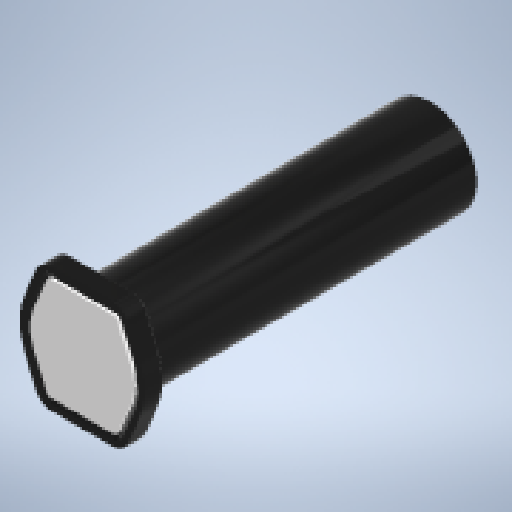
# Autodesk Inventor part: Spool Stud
Saved by Autodesk Inventor 2024 (Build 280153000, 153)
## iProperties
Created: 2025-01-02
Part Number: Spool Stud
Material: ABS Plastic
Document SubType Name: Modeling
Designer: Ishaan
Density: 1.06 g/cm^3
Appearance: Smooth - Black
Author: Ishaan
Autodesk Inventor part; units mm, degrees
ref_plane "YZ Plane" through (0, 0, 0) normal (1, 0, 0) x (0, 1, 0)
ref_plane "XZ Plane" through (0, 0, 0) normal (0, 1, 0) x (-1, 0, 0)
ref_plane "XY Plane" through (0, 0, 0) normal (0, 0, 1) x (1, 0, 0)
sketch "Sketch1" plane through (0, 0, 0) normal (0, 0, 1) x (1, 0, 0)
  circle A0 centre (0, 0) radius 15
  dimension "d0" = 30
  constraints: 1 centre point, 1 coincident
  measures "d0" diameter of A0
extrude "Extrusion1" add sketch "Sketch1" along normal blind 105
ref_plane "Work Plane1" through (0, 0, 8) normal (0, 0, -1) x (-1, 0, 0)
sketch "Sketch2" plane through (0, 0, 105) normal (0, 0, 1) x (1, 0, 0)
  line L0 (0, 7.5) -> (0, -7.5) construction
  point P0 (0, 0)
  point P1 (0, 0)
  dimension "d4" = 15
  constraints: 2 end point, 1 coincident, 1 midpoint, 1 vertical
  measures "d4" distance of L0.start L0.end
hole "Hole1" at (0, 7.5, 105) at (0, -7.5, 105) direction (0, 0, -1) diameter 10 depth 97
sketch "Sketch3" plane through (0, 7.5, 8) normal (0, 0, 1) x (1, 0, 0)
  circle A0 centre (0, 0) radius 5 projected
  circle A1 centre (0, -15) radius 5 projected
  point P0 (0, -7.5)
hole "Hole2" at (0, 7.5, 8) at (0, -7.5, 8) direction (0, 0, -1) diameter 5.4 end through all
sketch "Sketch4" plane through (0, 0, 105) normal (0, 0, 1) x (1, 0, 0)
  circle A0 centre (0, -7.5) radius 5 projected
  circle A1 centre (0, 7.5) radius 5 projected
  circle A2 centre (0, 0) radius 15 projected
  circle A3 centre (0, 0) radius 20
  line L0 (-18.4776, 7.6537) -> (-13.3636, 20)
  line L1 (-13.3636, 20) -> (13.3636, 20)
  line L2 (13.3636, 20) -> (18.4776, 7.6537)
  line L3 (18.4776, -7.6537) -> (13.3636, -20)
  line L4 (13.3636, -20) -> (-13.3636, -20)
  line L5 (-13.3636, -20) -> (-18.4776, -7.6537)
  dimension "d19" = 40
  dimension "d20" = 135
  dimension "d21" = 135
  constraints: 12 end point, 6 tangent, 4 point on circle, 2 horizontal, 2 vertical alignment, 1 centre point, 1 coincident
  measures "d19" diameter of A3
  measures "d20" angle of L3 L2
  measures "d21" angle of L5 L0
extrude "Extrusion2" add sketch "Sketch4" along normal blind 6.5 contours A2 | A3 | A3 L1 L2 | L3 L4 A3 | A3 L0 L1 | L4 L5 A3
fillet "Fillet1" radius 5 4 edges at (-13.3636, 20, 108.25) (-13.3636, -20, 108.25) (13.3636, -20, 108.25) (13.3636, 20, 108.25)
sketch "Sketch5" plane through (0, 0, 111.5) normal (0, 0, 1) x (1, 0, 0)
  arc A0 (14.6421, 16.9134) -> (10.0227, 20) centre (10.0227, 15) ccw projected
  line L0 (10.0227, 20) -> (-10.0227, 20) projected
  arc A1 (-10.0227, 20) -> (-14.6421, 16.9134) centre (-10.0227, 15) ccw projected
  line L1 (-14.6421, 16.9134) -> (-18.4776, 7.6537) projected
  arc A2 (-18.4776, 7.6537) -> (-18.4776, -7.6537) centre (0, 0) ccw projected
  line L2 (-18.4776, -7.6537) -> (-14.6421, -16.9134) projected
  arc A3 (-14.6421, -16.9134) -> (-10.0227, -20) centre (-10.0227, -15) ccw projected
  line L3 (-10.0227, -20) -> (10.0227, -20) projected
  arc A4 (10.0227, -20) -> (14.6421, -16.9134) centre (10.0227, -15) ccw projected
  line L4 (14.6421, -16.9134) -> (18.4776, -7.6537) projected
  arc A5 (18.4776, -7.6537) -> (18.4776, 7.6537) centre (0, 0) ccw projected
  line L5 (18.4776, 7.6537) -> (14.6421, 16.9134) projected
  circle A6 centre (0, 7.5) radius 5 projected
  circle A7 centre (0, -7.5) radius 5 projected
  line L6 (-10.0227, 18) -> (10.0227, 18)
  arc A8 (12.7943, 16.1481) -> (10.0227, 18) centre (10.0227, 15) ccw
  line L7 (12.7943, 16.1481) -> (16.6298, 6.8883)
  arc A9 (16.6298, -6.8883) -> (16.6298, 6.8883) centre (0, 0) ccw
  line L8 (16.6298, -6.8883) -> (12.7943, -16.1481)
  arc A10 (10.0227, -18) -> (12.7943, -16.1481) centre (10.0227, -15) ccw
  line L9 (10.0227, -18) -> (-10.0227, -18)
  arc A11 (-12.7943, -16.1481) -> (-10.0227, -18) centre (-10.0227, -15) ccw
  line L10 (-12.7943, -16.1481) -> (-16.6298, -6.8883)
  arc A12 (-16.6298, 6.8883) -> (-16.6298, -6.8883) centre (0, 0) ccw
  line L11 (-16.6298, 6.8883) -> (-12.7943, 16.1481)
  arc A13 (-10.0227, 18) -> (-12.7943, 16.1481) centre (-10.0227, 15) ccw
  dimension "d25" = 2
  constraints: 12 end point, 12 point on circle, 6 centre point, 11 other
  measures "d25" distance between parallel lines of L0 L6
extrude "Extrusion3" cut sketch "Sketch5" against normal blind 2.5 contours L6 A8 L7 A9 L8 A10 L9 A11 L10 A12 L11 A13
chamfer "Chamfer1" distance 2.5 angle 45 12 edges at (-14.7121, 11.5182, 109) (-11.6894, 17.4944, 109) (0, 18, 109) (11.6894, 17.4944, 109) (14.7121, 11.5182, 109) (18, 0, 109) (14.7121, -11.5182, 109) (11.6894, -17.4944, 109) (0, -18, 109) (-11.6894, -17.4944, 109) (-14.7121, -11.5182, 109) (-18, 0, 109)
ref_plane "Work Plane2" through (0, 0, 109.4) normal (0, 0, 1) x (1, 0, 0)
sketch "Sketch6" plane through (0, 0, 109) normal (0, 0, 1) x (1, 0, 0)
  circle A0 centre (0, 7.5) radius 5 projected
  circle A1 centre (0, -7.5) radius 5 projected
  line L0 (-14.3201, 5.9316) -> (-10.4846, 15.1913) projected
  arc A2 (-14.3201, 5.9316) -> (-14.3201, -5.9316) centre (0, 0) ccw projected
  line L1 (-10.4846, -15.1913) -> (-14.3201, -5.9316) projected
  arc A3 (-10.4846, -15.1913) -> (-10.0227, -15.5) centre (-10.0227, -15) ccw projected
  line L2 (10.0227, -15.5) -> (-10.0227, -15.5) projected
  arc A4 (10.0227, -15.5) -> (10.4846, -15.1913) centre (10.0227, -15) ccw projected
  line L3 (14.3201, -5.9316) -> (10.4846, -15.1913) projected
  arc A5 (14.3201, -5.9316) -> (14.3201, 5.9316) centre (0, 0) ccw projected
  line L4 (10.4846, 15.1913) -> (14.3201, 5.9316) projected
  arc A6 (10.4846, 15.1913) -> (10.0227, 15.5) centre (10.0227, 15) ccw projected
  line L5 (-10.0227, 15.5) -> (10.0227, 15.5) projected
  arc A7 (-10.0227, 15.5) -> (-10.4846, 15.1913) centre (-10.0227, 15) ccw projected
  arc A8 (11.4085, 15.574) -> (10.0227, 16.5) centre (10.0227, 15) ccw
  line L6 (11.4085, 15.574) -> (15.244, 6.3143)
  arc A9 (15.244, -6.3143) -> (15.244, 6.3143) centre (0, 0) ccw
  line L7 (15.244, -6.3143) -> (11.4085, -15.574)
  arc A10 (10.0227, -16.5) -> (11.4085, -15.574) centre (10.0227, -15) ccw
  line L8 (10.0227, -16.5) -> (-10.0227, -16.5)
  arc A11 (-11.4085, -15.574) -> (-10.0227, -16.5) centre (-10.0227, -15) ccw
  line L9 (-11.4085, -15.574) -> (-15.244, -6.3143)
  arc A12 (-15.244, 6.3143) -> (-15.244, -6.3143) centre (0, 0) ccw
  line L10 (-15.244, 6.3143) -> (-11.4085, 15.574)
  arc A13 (-10.0227, 16.5) -> (-11.4085, 15.574) centre (-10.0227, 15) ccw
  line L11 (-10.0227, 16.5) -> (10.0227, 16.5)
  dimension "d31" = 1
  constraints: 12 end point, 12 point on circle, 6 centre point, 11 other
  measures "d31" distance between parallel lines of L5 L11
extrude "Extrusion4" add sketch "Sketch6" along normal up to surface (2.1 mm away) from surface at 0.4 separate body contours A0 | A1 | L0 A7 L5 A6 L4 A5 L3 A4 L2 A3 L1 A2 | L6 A9 L7 A10 L8 A11 L9 A12 L10 A13 L11 A8
chamfer "Chamfer2" distance 1.25 angle 45 12 edges at (0, 16.5, 109.4) (10.856, 16.2472, 109.4) (13.3263, 10.9442, 109.4) (16.5, 0, 109.4) (13.3263, -10.9442, 109.4) (10.856, -16.2472, 109.4) (0, -16.5, 109.4) (-10.856, -16.2472, 109.4) (-13.3263, -10.9442, 109.4) (-16.5, 0, 109.4) (-13.3263, 10.9442, 109.4) (-10.856, 16.2472, 109.4)
sketch "Sketch7" plane through (0, 0, 109.4) normal (0, 0, -1) x (-1, 0, 0)
  arc A0 (-14.6421, -16.9134) -> (-10.0227, -20) centre (-10.0227, -15) ccw projected
  line L0 (-14.6421, -16.9134) -> (-18.4776, -7.6537) projected
  arc A1 (-18.4776, 7.6537) -> (-18.4776, -7.6537) centre (0, 0) ccw projected
  line L1 (-18.4776, 7.6537) -> (-14.6421, 16.9134) projected
  arc A2 (-10.0227, 20) -> (-14.6421, 16.9134) centre (-10.0227, 15) ccw projected
  line L2 (-10.0227, 20) -> (10.0227, 20) projected
  arc A3 (14.6421, 16.9134) -> (10.0227, 20) centre (10.0227, 15) ccw projected
  line L3 (14.6421, 16.9134) -> (18.4776, 7.6537) projected
  arc A4 (18.4776, -7.6537) -> (18.4776, 7.6537) centre (0, 0) ccw projected
  line L4 (18.4776, -7.6537) -> (14.6421, -16.9134) projected
  arc A5 (10.0227, -20) -> (14.6421, -16.9134) centre (10.0227, -15) ccw projected
  line L5 (10.0227, -20) -> (-10.0227, -20) projected
  circle A6 centre (0, 7.5) radius 4.7
  circle A7 centre (0, -7.5) radius 4.7
  line L6 (14.6897, 6.0847) -> (10.8542, 15.3444) projected
  arc A8 (10.8542, 15.3444) -> (10.0227, 15.9) centre (10.0227, 15) ccw projected
  line L7 (10.0227, 15.9) -> (-10.0227, 15.9) projected
  arc A9 (-10.0227, 15.9) -> (-10.8542, 15.3444) centre (-10.0227, 15) ccw projected
  line L8 (-10.8542, 15.3444) -> (-14.6897, 6.0847) projected
  arc A10 (-14.6897, 6.0847) -> (-14.6897, -6.0847) centre (0, 0) ccw projected
  line L9 (-14.6897, -6.0847) -> (-10.8542, -15.3444) projected
  arc A11 (-10.8542, -15.3444) -> (-10.0227, -15.9) centre (-10.0227, -15) ccw projected
  line L10 (-10.0227, -15.9) -> (10.0227, -15.9) projected
  arc A12 (10.0227, -15.9) -> (10.8542, -15.3444) centre (10.0227, -15) ccw projected
  line L11 (10.8542, -15.3444) -> (14.6897, -6.0847) projected
  arc A13 (14.6897, -6.0847) -> (14.6897, 6.0847) centre (0, 0) ccw projected
  line L12 (-10.0227, 15.25) -> (10.0227, 15.25) projected
  arc A14 (10.2536, 15.0957) -> (10.0227, 15.25) centre (10.0227, 15) ccw projected
  line L13 (10.2536, 15.0957) -> (14.0892, 5.8359) projected
  arc A15 (14.0892, -5.8359) -> (14.0892, 5.8359) centre (0, 0) ccw projected
  line L14 (14.0892, -5.8359) -> (10.2536, -15.0957) projected
  arc A16 (10.0227, -15.25) -> (10.2536, -15.0957) centre (10.0227, -15) ccw projected
  line L15 (10.0227, -15.25) -> (-10.0227, -15.25) projected
  arc A17 (-10.2536, -15.0957) -> (-10.0227, -15.25) centre (-10.0227, -15) ccw projected
  line L16 (-10.2536, -15.0957) -> (-14.0892, -5.8359) projected
  arc A18 (-14.0892, 5.8359) -> (-14.0892, -5.8359) centre (0, 0) ccw projected
  line L17 (-14.0892, 5.8359) -> (-10.2536, 15.0957) projected
  arc A19 (-10.0227, 15.25) -> (-10.2536, 15.0957) centre (-10.0227, 15) ccw projected
  constraints: 2 centre point, 1 equal radius
extrude "Extrusion5" add sketch "Sketch7" along normal blind 6 contours A6 | A7 bodies 2
fillet "Fillet2" radius 1 2 edges at (4.7, 7.5, 103.4) (4.7, -7.5, 103.4)
fillet "Fillet3" radius 0.5 2 edges at (4.7, 7.5, 109.4) (4.7, -7.5, 109.4)
fillet "Fillet4" radius 0.5 2 edges at (-5, -7.5, 109) (-5, 7.5, 109)
sketch "Sketch8" plane through (0, 0, 0) normal (1, 0, 0) x (0, 1, 0)
  line L0 (-10.2, 8) -> (-10.2, 0) projected
  line L1 (-10.2, 0) -> (-15, 0) projected
  line L2 (-15, 0) -> (-15, 105) projected
  line L3 (-15, 105) -> (-20, 105) projected
  line L4 (-20, 105) -> (-20, 111.5) projected
  line L5 (-20, 111.5) -> (-18, 111.5) projected
  line L6 (-18, 111.5) -> (-15.5, 109) projected
  line L7 (-15.5, 109) -> (-13, 109) projected
  arc A0 (-12.5, 108.5) -> (-13, 109) centre (-13, 108.5) ccw projected
  line L8 (-12.5, 108.5) -> (-12.5, 8) projected
  line L9 (-12.5, 8) -> (-10.2, 8) projected
  line L10 (10.2, 0) -> (10.2, 8) projected
  line L11 (10.2, 8) -> (12.5, 8) projected
  line L12 (12.5, 8) -> (12.5, 108.5) projected
  arc A1 (13, 109) -> (12.5, 108.5) centre (13, 108.5) ccw projected
  line L13 (13, 109) -> (15.5, 109) projected
  line L14 (15.5, 109) -> (18, 111.5) projected
  line L15 (18, 111.5) -> (20, 111.5) projected
  line L16 (20, 111.5) -> (20, 105) projected
  line L17 (20, 105) -> (15, 105) projected
  line L18 (15, 105) -> (15, 0) projected
  line L19 (15, 0) -> (10.2, 0) projected
  line L20 (4.8, 8) -> (4.8, 0) projected
  line L21 (4.8, 0) -> (-4.8, 0) projected
  line L22 (-4.8, 0) -> (-4.8, 8) projected
  line L23 (-4.8, 8) -> (-2.5, 8) projected
  line L24 (-2.5, 8) -> (-2.5, 108.5) projected
  arc A2 (-2, 109) -> (-2.5, 108.5) centre (-2, 108.5) ccw projected
  line L25 (-2, 109) -> (2, 109) projected
  arc A3 (2.5, 108.5) -> (2, 109) centre (2, 108.5) ccw projected
  line L26 (2.5, 108.5) -> (2.5, 8) projected
  line L27 (2.5, 8) -> (4.8, 8) projected
  line L28 (15.25, 109.4) -> (12.7, 109.4) projected
  arc A4 (12.7, 109.4) -> (12.2, 108.9) centre (12.7, 108.9) ccw projected
  line L29 (12.2, 108.9) -> (12.2, 104.4) projected
  arc A5 (11.2, 103.4) -> (12.2, 104.4) centre (11.2, 104.4) ccw projected
  line L30 (11.2, 103.4) -> (3.8, 103.4) projected
  arc A6 (2.8, 104.4) -> (3.8, 103.4) centre (3.8, 104.4) ccw projected
  line L31 (2.8, 104.4) -> (2.8, 108.9) projected
  arc A7 (2.8, 108.9) -> (2.3, 109.4) centre (2.3, 108.9) ccw projected
  line L32 (2.3, 109.4) -> (-2.3, 109.4) projected
  arc A8 (-2.3, 109.4) -> (-2.8, 108.9) centre (-2.3, 108.9) ccw projected
  line L33 (-2.8, 108.9) -> (-2.8, 104.4) projected
  arc A9 (-3.8, 103.4) -> (-2.8, 104.4) centre (-3.8, 104.4) ccw projected
  line L34 (-3.8, 103.4) -> (-11.2, 103.4) projected
  arc A10 (-12.2, 104.4) -> (-11.2, 103.4) centre (-11.2, 104.4) ccw projected
  line L35 (-12.2, 104.4) -> (-12.2, 108.9) projected
  arc A11 (-12.2, 108.9) -> (-12.7, 109.4) centre (-12.7, 108.9) ccw projected
  line L36 (-12.7, 109.4) -> (-15.25, 109.4) projected
  line L37 (-15.25, 109.4) -> (-16.5, 110.65) projected
  line L38 (-16.5, 110.65) -> (-16.5, 111.5) projected
  line L39 (-16.5, 111.5) -> (16.5, 111.5) projected
  line L40 (16.5, 111.5) -> (16.5, 110.65) projected
  line L41 (16.5, 110.65) -> (15.25, 109.4) projected
  circle A12 centre (2.8, 105.5) radius 0.55
  circle A13 centre (2.8, 105.5) radius 0.4
  line L42 (2.8, 105.9) -> (2.8, 105.1)
  line L43 (2.8, 106.05) -> (2.8, 104.95)
  point P0 (0, 0)
  dimension "d45" = 3.5
  dimension "d46" = 0.8
  dimension "d47" = 0.15
  constraints: 5 point on line, 4 end point, 4 point on circle, 2 centre point, 1 coincident
  measures "d45" distance from line of A12.centre L25
  measures "d46" diameter of A13
  measures "d47" radial gap between concentric circles of A12 A13
revolve "Revolution1" cut sketch "Sketch8" angle 360 about axis through (0, 2.8, 104.4) along (0, 0, 1) bodies 1 contours A12 L26 A13 | L26 A13 L31 A12 | A13 L26 | L26 A13 L31 | A12 L31 A13 L26
revolve "Revolution2" add sketch "Sketch8" angle 360 about axis through (0, 2.8, 106.05) along (0, 0, -1) bodies 2 contours A13 L26 | L26 A13 L31
fillet "Fillet5" radius 0.5 2 edges at (-0.4749, 2.5226, 105.5002) (0.4749, 2.5226, 105.4999)
fillet "Fillet6" radius 0.5 2 edges at (0.3996, 2.817, 105.4991) (-0.3996, 2.817, 105.5)
mirror "Mirror1" about plane through (0, 0, 0) normal (0, 1, 0) of "Revolution1", "Fillet5" bodies 1
mirror "Mirror2" about plane through (0, 0, 0) normal (0, 1, 0) of "Revolution2", "Fillet6" bodies 2
fillet "Fillet7" radius 1 1 edges at (-15, 0, 105)
fillet "Fillet8" radius 1 12 edges at (-12.8005, 19.1573, 105) (-16.5598, 12.2835, 105) (-20, 0, 105) (-16.5598, -12.2835, 105) (-12.8005, -19.1573, 105) (0, -20, 105) (12.8005, -19.1573, 105) (16.5598, -12.2835, 105) (20, 0, 105) (16.5598, 12.2835, 105) (12.8005, 19.1573, 105) (0, 20, 105)
equation "\"d21\" = d20"
body "Solid1"
body "Solid2"
